Autodesk Fusion 360 part; units mm, degrees
(part 5 of 5)
sketch "Sketch5" plane through (0, 0, -6) normal (0, 0, -1) x (1, 0, 0)
  line L0 (373.812, -103.824) -> (373.812, -106.4798)
  line L1 (373.812, -106.4798) -> (371.512, -107.8077)
  line L2 (371.512, -107.8077) -> (369.212, -106.4798)
  line L3 (369.212, -106.4798) -> (369.212, -103.824)
  line L4 (369.212, -103.824) -> (371.512, -102.4961)
  line L5 (371.512, -102.4961) -> (373.812, -103.824)
  line L6 (373.812, 5.5979) -> (373.812, 2.9421)
  line L7 (373.812, 2.9421) -> (371.512, 1.6142)
  line L8 (371.512, 1.6142) -> (369.212, 2.9421)
  line L9 (369.212, 2.9421) -> (369.212, 5.5979)
  line L10 (369.212, 5.5979) -> (371.512, 6.9258)
  line L11 (371.512, 6.9258) -> (373.812, 5.5979)
  line L12 (-2.3103, 5.5979) -> (-2.3103, 2.9421)
  line L13 (-2.3103, 2.9421) -> (-4.6104, 1.6142)
  line L14 (-4.6104, 1.6142) -> (-6.9103, 2.9421)
  line L15 (-6.9103, 2.9421) -> (-6.9103, 5.5979)
  line L16 (-6.9103, 5.5979) -> (-4.6104, 6.9258)
  line L17 (-4.6104, 6.9258) -> (-2.3103, 5.5979)
  line L18 (-2.3103, -103.824) -> (-2.3103, -106.4798)
  line L19 (-2.3103, -106.4798) -> (-4.6104, -107.8077)
  line L20 (-4.6104, -107.8077) -> (-6.9103, -106.4798)
  line L21 (-6.9103, -106.4798) -> (-6.9103, -103.824)
  line L22 (-6.9103, -103.824) -> (-4.6104, -102.4961)
  line L23 (-4.6104, -102.4961) -> (-2.3103, -103.824)
  line L24 (169.4884, -103.1519) -> (169.4884, -113.1519)
  line L25 (169.4884, -113.1519) -> (371.512, -113.1519)
  arc A0 (371.512, -113.1519) -> (379.512, -105.1519) centre (371.512, -105.1519) ccw
  line L26 (379.512, -105.1519) -> (379.512, 4.27)
  arc A1 (379.512, 4.27) -> (371.512, 12.27) centre (371.512, 4.27) ccw
  line L27 (371.512, 12.27) -> (-4.6103, 12.27)
  arc A2 (-4.6104, 12.27) -> (-12.6103, 4.27) centre (-4.6103, 4.27) ccw
  line L28 (-12.6103, 4.27) -> (-12.6103, -105.1519)
  arc A3 (-12.6103, -105.1519) -> (-4.6103, -113.1519) centre (-4.6103, -105.1519) ccw
  line L29 (-4.6103, -113.1519) -> (154.4884, -113.1519)
  line L30 (154.4884, -113.1519) -> (154.4884, -103.1519)
  line L31 (154.4884, -103.1519) -> (1.3896, -103.1519)
  arc A4 (-2.6103, -99.1519) -> (1.3896, -103.1519) centre (1.3897, -99.1519) ccw
  line L32 (-2.6103, -99.1519) -> (-2.6103, -1.73)
  arc A5 (1.3897, 2.27) -> (-2.6103, -1.73) centre (1.3897, -1.73) ccw
  line L33 (1.3897, 2.27) -> (365.512, 2.27)
  arc A6 (369.512, -1.73) -> (365.512, 2.27) centre (365.512, -1.73) ccw
  line L34 (369.512, -1.73) -> (369.512, -99.1519)
  arc A7 (365.512, -103.1519) -> (369.512, -99.1519) centre (365.512, -99.1519) ccw
  line L35 (365.512, -103.1519) -> (169.4884, -103.1519)
  circle A8 centre (371.512, -105.1519) radius 1.55
  circle A9 centre (371.512, 4.27) radius 1.55
  circle A10 centre (-4.6103, 4.27) radius 1.55
  circle A11 centre (-4.6103, -105.1519) radius 1.55
  arc A12 (-12.6103, -105.1519) -> (-4.6103, -113.1519) centre (-4.6103, -105.1519) ccw
  line L36 (-12.6103, 4.27) -> (-12.6103, -105.1519)
  line L37 (-4.6103, -113.1519) -> (371.512, -113.1519)
  arc A13 (371.512, -113.1519) -> (379.512, -105.1519) centre (371.512, -105.1519) ccw
  line L38 (379.512, -105.1519) -> (379.512, 4.27)
  arc A14 (379.512, 4.27) -> (371.512, 12.27) centre (371.512, 4.27) ccw
  line L39 (371.512, 12.27) -> (-4.6103, 12.27)
  arc A15 (-4.6104, 12.27) -> (-12.6103, 4.27) centre (-4.6103, 4.27) ccw
  line L40 (169.4884, -113.1519) -> (169.4884, -108.1519)
  line L41 (169.4884, -108.1519) -> (154.4884, -108.1519)
  line L42 (154.4884, -108.1519) -> (154.4884, -113.1519)
  constraint vertical L40
  constraint horizontal L41
  constraint vertical L42
  constraint midpoint L24 L40.end
  constraint coincident L29.end L30.start
extrude "Extrude4" add sketch "Sketch5" along normal blind 3 separate body contours L0 L1 L2 L3 L4 L5 | L6 L7 L8 L9 L10 L11 | L12 L13 L14 L15 L16 L17 | L18 L19 L20 L21 L22 L23 | L24 L25 A0 L26 A1 L27 A2 L28 A3 L29 L30 L31 A4 L32 A5 L33 A6 L34 A7 L35 A12 L36 L37 A13 L38 A14 L39 A15 L40 L42 | L24 L30 L31 A4 L32 A5 L33 A6 L34 A7 L35 L41 makes body 3
equation "d32 = ( 4.6 / 2 ) * 1 mm"
